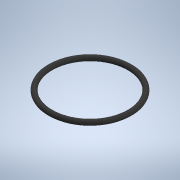
# Autodesk Inventor part: 2-023
Saved by Autodesk Inventor 2021 (Build 250183000, 183)
## iProperties
Created: 2021-10-18
Part Number: 2-023
Material: Rubber
Document SubType Name: Modeling
Designer: Alex Clay
Density: 0.93 g/cm^3
Appearance: Rubber - Black
Mass: 0.206366 g
Surface Area: 4.9921 cm^2
Volume: 0.221899 cm^3
Author: ALEX CLAY
Comments: PARKER SIZE 2-023
Autodesk Inventor part; units mm, degrees
ref_plane "YZ Plane" through (0, 0, 0) normal (1, 0, 0) x (0, 1, 0)
ref_plane "XZ Plane" through (0, 0, 0) normal (0, 1, 0) x (-1, 0, 0)
ref_plane "XY Plane" through (0, 0, 0) normal (0, 0, 1) x (1, 0, 0)
sketch "Sketch1" plane through (0, 0, 0) normal (0, 0, 1) x (1, 0, 0)
  circle A0 centre (14.224, 0) radius 0.889
  line L0 (13.335, 5.9933) -> (13.335, -5.58) construction
  line L1 (-3.0226, 0) -> (18.1356, 0) projected
  line L2 (0, -7.8947) -> (0, 8.308) projected
  point P0 (0, 0)
  dimension "d0" = 1.778
  dimension "d1" = 13.335
  constraints: 2 end point, 1 centre point, 1 point on line, 1 tangent, 1 vertical
  measures "d0" diameter of A0
  measures "d1" distance from line of point (0, 0) L0
revolve "Revolution1" add sketch "Sketch1" angle 360 about axis through (0, -10, 0) along (0, 1, 0)
body "Solid1"
